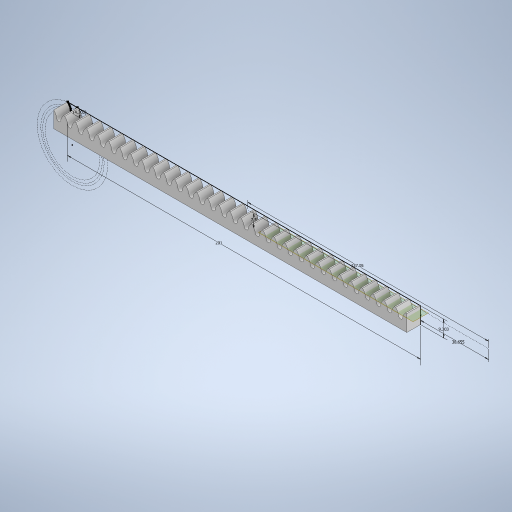
# Autodesk Inventor part: pinion_V2
Saved by Autodesk Inventor 2023 (Build 270158000, 158)
## iProperties
Created: 2022-11-22
Part Number: pinion_V2
Material: Generic
Document SubType Name: Modeling
Designer: shrey
Density: 1 g/cm^3
Appearance: Default
Author: shrey
Autodesk Inventor part; units mm, degrees
ref_plane "YZ Plane" through (0, 0, 0) normal (1, 0, 0) x (0, 1, 0)
ref_plane "XZ Plane" through (0, 0, 0) normal (0, 1, 0) x (-1, 0, 0)
ref_plane "XY Plane" through (0, 0, 0) normal (0, 0, 1) x (1, 0, 0)
sketch "Sketch1" plane through (0, 0, 0) normal (0, 0, 1) x (1, 0, 0)
  spline S0 degree 3 poles (-2.798, 19.8033) (-2.6544, 19.6281) (-2.3672, 19.2776) (-1.9857, 18.7145) (-1.6476, 18.1243) (-1.4193, 17.6053) (-1.275, 17.175) (-1.2174, 16.8397) (-1.1733, 16.5031) (-1.0767, 16.1754) (-0.9083, 15.8767) (-0.6621, 15.6364) (-0.3416, 15.4963) (0, 15.5019) (0.3416, 15.4963) (0.6621, 15.6364) (0.9083, 15.8767) (1.0767, 16.1754) (1.1733, 16.5031) (1.2174, 16.8397) (1.275, 17.175) (1.4193, 17.6053) (1.6476, 18.1243) (1.9857, 18.7145) (2.3672, 19.2776) (2.6544, 19.6281) (2.798, 19.8033) knots 0 0 0 0 0.067937 0.135874 0.203802 0.271714 0.30568 0.339609 0.373555 0.407503 0.441435 0.475301 0.509129 0.543019 0.576909 0.610738 0.644604 0.678536 0.712484 0.74643 0.780359 0.814325 0.882236 0.950165 1.018102 1.086039 1.086039 1.086039 1.086039
  circle A0 centre (0, 0) radius 15.5 construction
  circle A1 centre (0, 0) radius 16.9145 construction
  circle A2 centre (0, 0) radius 18 construction
  circle A3 centre (0, 0) radius 20 construction
  line L0 (-2.798, 19.8033) -> (2.798, 19.8033)
  line L1 (-2.798, 19.8033) -> (198.202, 19.8033)
  line L2 (198.202, 19.8033) -> (198.202, 10.5003)
  line L3 (198.202, 10.5003) -> (-2.798, 10.5003)
  line L4 (-2.798, 10.5003) -> (-2.798, 19.8033)
  line L5 (99.8068, 18) -> (236.857, 18) construction
  point P0 (-2.3754, 19.2714)
  point P1 (-1.9929, 18.7099)
  point P2 (-1.6582, 18.1188)
  point P3 (-1.3864, 17.4965)
  point P4 (-1.2834, 17.1728)
  point P5 (-1.2197, 16.8395)
  point P6 (-1.1646, 16.5046)
  point P7 (-1.0647, 16.1801)
  point P8 (-0.8952, 15.8862)
  point P9 (-0.6496, 15.653)
  point P10 (-0.3383, 15.5206)
  point P11 (0, 15.5)
  point P12 (0.3383, 15.5206)
  point P13 (0.6496, 15.653)
  point P14 (0.8952, 15.8862)
  point P15 (1.0647, 16.1801)
  point P16 (1.1646, 16.5046)
  point P17 (1.2197, 16.8395)
  point P18 (1.2834, 17.1728)
  point P19 (1.3864, 17.4965)
  point P20 (1.6582, 18.1188)
  point P21 (1.9929, 18.7099)
  point P22 (2.3754, 19.2714)
  point P23 (198.202, 15.1518)
  dimension "d2" = 9.303
  dimension "d3" = 201
  dimension "d4" = 4.3033
  dimension "d12" = 137.0502
  dimension "d15" = 38.655
  dimension "d16" = 7.4997
  constraints: 12 end point, 4 centre point, 4 horizontal, 2 parallel, 2 point on circle, 2 point on line, 1 midpoint, 1 perpendicular, 55 other
  measures "d2" distance of L1.end L2.end
  measures "d3" distance of L2.end L3.end
  measures "d4" vertical distance of L0.end point (0, 15.5)
  measures "d12" distance of L5.start L5.end
  measures "d15" horizontal distance of point (198.202, 15.152) L5.end
  measures "d16" distance between parallel lines of L3 L5
extrude "Extrusion2" add sketch "Sketch1" along normal blind 7.82
extrude "Extrusion3" cut sketch "Sketch1" along normal through all contours L0 S0
pattern_linear "Rectangular Pattern1" count 32 spacing 6.28 along (1, 0, 0) of "Extrusion3"
ref_plane "Work Plane1" through (99.8068, 18, 0) normal (0, -1, 0) x (1, 0, 0)
equation "\"Module\" = 2"
equation "\"PressureAngle\" = 20deg"
equation "\"UnitProfileClearance\" = 0.25"
equation "\"UnitRoundRadius\" = 0.35"
equation "\"RootDiameter\" = 31"
equation "\"BaseDiameter\" = 33.82893"
equation "\"PitchDiameter\" = 36"
equation "\"HelixAngle\" = 0"
equation "\"UnitCorrection\" = 0"
equation "\"UnitAddendumModification\" = 0"
equation "\"CircularPitch\" = 6.283185"
equation "\"UnitBacklashShift\" = 0"
equation "\"TotalToolShift\" = 0"
equation "\"IsInternal\" = 0"
